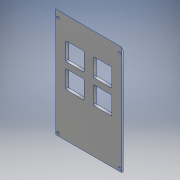
# Autodesk Inventor part: front_cover
Saved by Autodesk Inventor 2016 (Build 200138000, 138)
## iProperties
Created: 2017-09-09
Part Number: front_cover
Material: Aluminum 6061
Document SubType Name: Modeling
Designer: Davide
Density: 2.7 g/cm^3
Appearance: Aluminum - Flat
Mass: 35.662 g
Surface Area: 185.696 cm^2
Volume: 13.2082 cm^3
Author: Davide
Autodesk Inventor part; units mm, degrees
ref_plane "YZ Plane" through (0, 0, 0) normal (1, 0, 0) x (0, 1, 0)
sketch "Sketch1" plane through (0, 0, 0) normal (0, 1, 0) x (-1, 0, 0)
  line L0 (38, 60.75) -> (-38, 60.75)
  line L1 (-38, 60.75) -> (-38, -60.75)
  line L2 (-38, -60.75) -> (38, -60.75)
  line L3 (38, -60.75) -> (38, 60.75)
  line L4 (0, 60.75) -> (0, -60.75) construction
  line L5 (-6.5, 39.25) -> (-25.5, 39.25)
  line L6 (-26.5, 38.25) -> (-26.5, 19.25)
  line L7 (-25.5, 18.25) -> (-6.5, 18.25)
  line L8 (-5.5, 19.25) -> (-5.5, 38.25)
  arc A0 (-5.5, 38.25) -> (-6.5, 39.25) centre (-6.5, 38.25) ccw
  arc A1 (-6.5, 18.25) -> (-5.5, 19.25) centre (-6.5, 19.25) ccw
  arc A2 (-26.5, 19.25) -> (-25.5, 18.25) centre (-25.5, 19.25) ccw
  arc A3 (-25.5, 39.25) -> (-26.5, 38.25) centre (-25.5, 38.25) ccw
  circle A4 centre (35.5, 57.65) radius 1
  circle A5 centre (-35.5, 57.65) radius 1
  line L9 (0, 0) -> (-51.842, 0) construction
  circle A6 centre (35.5, -57.75) radius 1
  circle A7 centre (-35.5, -57.75) radius 1
  line L10 (6.5, 39.25) -> (25.5, 39.25)
  line L11 (26.5, 38.25) -> (26.5, 19.25)
  line L12 (25.5, 18.25) -> (6.5, 18.25)
  line L13 (5.5, 19.25) -> (5.5, 38.25)
  arc A8 (6.5, 39.25) -> (5.5, 38.25) centre (6.5, 38.25) ccw
  arc A9 (5.5, 19.25) -> (6.5, 18.25) centre (6.5, 19.25) ccw
  arc A10 (25.5, 18.25) -> (26.5, 19.25) centre (25.5, 19.25) ccw
  arc A11 (26.5, 38.25) -> (25.5, 39.25) centre (25.5, 38.25) ccw
  line L14 (25.5, -9.75) -> (6.5, -9.75)
  arc A12 (25.5, -9.75) -> (26.5, -8.75) centre (25.5, -8.75) ccw
  arc A13 (5.5, -8.75) -> (6.5, -9.75) centre (6.5, -8.75) ccw
  arc A14 (-6.5, -9.75) -> (-5.5, -8.75) centre (-6.5, -8.75) ccw
  line L15 (-25.5, -9.75) -> (-6.5, -9.75)
  arc A15 (-26.5, -8.75) -> (-25.5, -9.75) centre (-25.5, -8.75) ccw
  line L16 (-6.5, 11.25) -> (-25.5, 11.25)
  line L17 (-26.5, 10.25) -> (-26.5, -8.75)
  line L18 (-5.5, -8.75) -> (-5.5, 10.25)
  arc A16 (-5.5, 10.25) -> (-6.5, 11.25) centre (-6.5, 10.25) ccw
  arc A17 (-25.5, 11.25) -> (-26.5, 10.25) centre (-25.5, 10.25) ccw
  line L19 (5.5, -8.75) -> (5.5, 10.25)
  line L20 (26.5, 10.25) -> (26.5, -8.75)
  arc A18 (6.5, 11.25) -> (5.5, 10.25) centre (6.5, 10.25) ccw
  line L21 (6.5, 11.25) -> (25.5, 11.25)
  arc A19 (26.5, 10.25) -> (25.5, 11.25) centre (25.5, 10.25) ccw
  point P0 (-26.5, 18.25)
  point P1 (-26.5, 39.25)
  point P2 (-5.5, 18.25)
  point P3 (26.5, 18.25)
  point P4 (26.5, 39.25)
  point P5 (5.5, 18.25)
  point P6 (26.5, -9.75)
  point P7 (5.5, -9.75)
  point P8 (-5.5, -9.75)
  point P9 (-26.5, -9.75)
  point P10 (-26.5, 11.25)
  point P11 (26.5, 11.25)
  dimension "d0" = 121.5
  dimension "d1" = 76
  dimension "d2" = 21
  dimension "d3" = 21
  dimension "d5" = 1
  dimension "d15" = 2
  dimension "d30" = 3.1
  dimension "d31" = 2.5
  dimension "d33" = 3
  dimension "d52" = 5.5
  dimension "d55" = 28
  dimension "d60" = 100
  dimension "d73" = 2.5
  dimension "d74" = 2.5
  dimension "d75" = 2.5
  constraints: 44 end point, 32 point on circle, 24 point on line, 20 centre point, 17 symmetric about line, 8 tangent, 4 midpoint, 4 parallel, 3 equal radius, 3 horizontal, 2 perpendicular, 2 vertical, 52 other
  measures "d0" distance of L2.end L0.start
  measures "d1" distance of L0.start L0.end
  measures "d2" distance of point (-5.5, 18.25) point (-26.5, 18.25)
  measures "d3" distance of point (-26.5, 18.25) point (-26.5, 39.25)
  measures "d5" radius of A0
  measures "d15" diameter of A4
  measures "d30" distance from line of L0 A4.centre
  measures "d31" distance from line of L3 A4.centre
  measures "d33" distance from line of L2 A6.centre
  measures "d52" distance between parallel lines of L4 L8
  measures "d55" distance of point (26.5, 18.25) point (26.5, -9.75)
  measures "d60" distance between parallel lines of L5 L2
  measures "d73" distance from line of A6.centre L3
  measures "d74" distance from line of L1 A7.centre
  measures "d75" distance from line of L1 A5.centre
extrude "Extrusion6" add sketch "Sketch1" along normal blind 1.6
hole "Hole3" at (-35.5, 0, 57.65) at (35.5, 0, 57.65) at (-35.5, 0, -57.75) at (35.5, 0, -57.75) direction (0, 1, 0) diameter 2 depth 8 tip angle 118 countersink diameter 3 countersink angle 90
ref_plane "Work Plane1" through (-38.5, 0, -61) normal (-1, 0, 0) x (0, 0, 1)
sketch "Sketch2" plane through (-38.5, 0, -61) normal (-1, 0, 0) x (0, 0, 1)
  line L0 (0, 0) -> (121.75, 0) projected
  line L1 (121.75, 0) -> (121.75, 1.6) projected
  line L2 (121.75, 1.6) -> (125.924, 0)
  line L3 (121.75, 0) -> (125.924, 0)
  point P0 (61, 0)
  point P1 (121.924, 0)
  constraints: 4 end point, 1 horizontal
ref_plane "Work Plane2" through (0, 1.5, 0) normal (0, 1, 0) x (1, 0, 0)
extrude "Extrusion8" add sketch "Sketch2" against normal up to surface (76.5 mm away)
sketch "Sketch4" plane through (0, 1.6, 0) normal (0, 1, 0) x (1, 0, 0)
  arc A0 (6.5, 9.75) -> (5.5, 8.75) centre (6.5, 8.75) ccw projected
  line L0 (6.5, 9.75) -> (25.5, 9.75) projected
  arc A1 (26.5, 8.75) -> (25.5, 9.75) centre (25.5, 8.75) ccw projected
  line L1 (26.5, 8.75) -> (26.5, -10.25) projected
  arc A2 (25.5, -11.25) -> (26.5, -10.25) centre (25.5, -10.25) ccw projected
  line L2 (25.5, -11.25) -> (6.5, -11.25) projected
  arc A3 (5.5, -10.25) -> (6.5, -11.25) centre (6.5, -10.25) ccw projected
  line L3 (5.5, -10.25) -> (5.5, 8.75) projected
  arc A4 (-5.5, 8.75) -> (-6.5, 9.75) centre (-6.5, 8.75) ccw projected
  line L4 (-5.5, 8.75) -> (-5.5, -10.25) projected
  arc A5 (-6.5, -11.25) -> (-5.5, -10.25) centre (-6.5, -10.25) ccw projected
  line L5 (-6.5, -11.25) -> (-25.5, -11.25) projected
  arc A6 (-26.5, -10.25) -> (-25.5, -11.25) centre (-25.5, -10.25) ccw projected
  line L6 (-26.5, -10.25) -> (-26.5, 8.75) projected
  arc A7 (-25.5, 9.75) -> (-26.5, 8.75) centre (-25.5, 8.75) ccw projected
  line L7 (-25.5, 9.75) -> (-6.5, 9.75) projected
  arc A8 (-5.5, -19.25) -> (-6.5, -18.25) centre (-6.5, -19.25) ccw projected
  line L8 (-5.5, -19.25) -> (-5.5, -38.25) projected
  arc A9 (-6.5, -39.25) -> (-5.5, -38.25) centre (-6.5, -38.25) ccw projected
  line L9 (-6.5, -39.25) -> (-25.5, -39.25) projected
  arc A10 (-26.5, -38.25) -> (-25.5, -39.25) centre (-25.5, -38.25) ccw projected
  line L10 (-26.5, -38.25) -> (-26.5, -19.25) projected
  arc A11 (-25.5, -18.25) -> (-26.5, -19.25) centre (-25.5, -19.25) ccw projected
  line L11 (-25.5, -18.25) -> (-6.5, -18.25) projected
  arc A12 (6.5, -18.25) -> (5.5, -19.25) centre (6.5, -19.25) ccw projected
  line L12 (6.5, -18.25) -> (25.5, -18.25) projected
  arc A13 (26.5, -19.25) -> (25.5, -18.25) centre (25.5, -19.25) ccw projected
  line L13 (26.5, -19.25) -> (26.5, -38.25) projected
  arc A14 (25.5, -39.25) -> (26.5, -38.25) centre (25.5, -38.25) ccw projected
  line L14 (25.5, -39.25) -> (6.5, -39.25) projected
  arc A15 (5.5, -38.25) -> (6.5, -39.25) centre (6.5, -38.25) ccw projected
  line L15 (5.5, -38.25) -> (5.5, -19.25) projected
  circle A16 centre (35.5, 57.75) radius 1 projected
  circle A17 centre (-35.5, 57.75) radius 1 projected
  circle A18 centre (35.5, -57.65) radius 1 projected
  circle A19 centre (-35.5, -57.65) radius 1 projected
  line L16 (-38, -60.75) -> (38, -60.75) projected
  line L17 (38, -60.75) -> (38, 60.75) projected
  line L18 (38, 60.75) -> (-38, 60.75) projected
  line L19 (-38, 60.75) -> (-38, -60.75) projected
  line L20 (6.5, -40.45) -> (25.5, -40.45)
  arc A20 (25.5, -40.45) -> (27.7, -38.25) centre (25.5, -38.25) ccw
  line L21 (27.7, -38.25) -> (27.7, -19.25)
  arc A21 (27.7, -19.25) -> (25.5, -17.05) centre (25.5, -19.25) ccw
  line L22 (25.5, -17.05) -> (6.5, -17.05)
  arc A22 (6.5, -17.05) -> (4.3, -19.25) centre (6.5, -19.25) ccw
  line L23 (4.3, -19.25) -> (4.3, -38.25)
  arc A23 (4.3, -38.25) -> (6.5, -40.45) centre (6.5, -38.25) ccw
  line L24 (6.5, -12.45) -> (25.5, -12.45)
  arc A24 (25.5, -12.45) -> (27.7, -10.25) centre (25.5, -10.25) ccw
  line L25 (27.7, -10.25) -> (27.7, 8.75)
  arc A25 (27.7, 8.75) -> (25.5, 10.95) centre (25.5, 8.75) ccw
  line L26 (25.5, 10.95) -> (6.5, 10.95)
  arc A26 (6.5, 10.95) -> (4.3, 8.75) centre (6.5, 8.75) ccw
  line L27 (4.3, 8.75) -> (4.3, -10.25)
  arc A27 (4.3, -10.25) -> (6.5, -12.45) centre (6.5, -10.25) ccw
  point P0 (0, 0)
  dimension "d69" = 1.2
  dimension "d70" = 1.2
  constraints: 16 end point, 16 point on circle, 8 centre point, 14 other
  measures "d69" distance between parallel lines of L14 L20
  measures "d70" distance between parallel lines of L2 L24
extrude "Extrusion9" add sketch "Sketch4" along normal blind 1.6 contours A23 L23 A22 L22 A21 L21 A20 L20 | A27 L27 A26 L26 A25 L25 A24 L24
mirror "Mirror1" about plane through (0, 0, 0) normal (1, 0, 0) of "Extrusion9"
equation "\"d2\" = d3"
equation "\"d3\" = 1.05 * button_side"
equation "\"d73\" = d31"
equation "\"button_side\" = 20"
body "Solid1"
